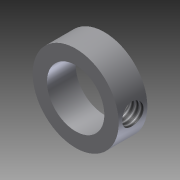
# Autodesk Inventor part: .5_inch_axle_bushing
Saved by Autodesk Inventor 2011 (Build 150239000, 239)
## iProperties
Created: 2013-01-17
Part Number: .5_inch_axle_bushing
Document SubType Name: Modeling
Designer: Christopher
Density: 1 g/cm^3
Author: Christopher
Autodesk Inventor part; units mm, degrees
ref_plane "YZ Plane" through (0, 0, 0) normal (1, 0, 0) x (0, 1, 0)
ref_plane "XZ Plane" through (0, 0, 0) normal (0, 1, 0) x (-1, 0, 0)
sketch "Sketch1" plane through (0, 0, 0) normal (0, 0, 1) x (1, 0, 0)
  circle A0 centre (0, 0) radius 6.35
  circle A1 centre (0, 0) radius 9.525
  point P0 (9.525, 0)
  dimension "d1" = 19.05
  dimension "d0" = 12.7
  constraints: 2 coincident, 1 centre point, 1 horizontal alignment, 2 other
  measures "d0" diameter of A0
extrude "Extrusion1" add sketch "Sketch1" against normal blind 6.35
ref_plane "Work Plane1" through (9.525, 0, 0) normal (1, 0, 0) x (0, 1, 0)
sketch "Sketch2" plane through (9.525, 0, 0) normal (1, 0, 0) x (0, 1, 0)
  line L0 (-9.525, 0) -> (9.525, 0) projected
  point P0 (0, 0)
  point P1 (0, -3.175)
  dimension "d4" = 3.175
  measures "d4" distance from line of L0 point (0, -3.175)
hole "Hole1" at (9.525, 0, -3.175) direction (-1, 0, 0) diameter 4.7625 depth 6.35 tip angle 118
thread "Thread1" size "10-24 UNC" class "2B" standard "ANSI Unified Screw Threads" full length
body "Solid1"
